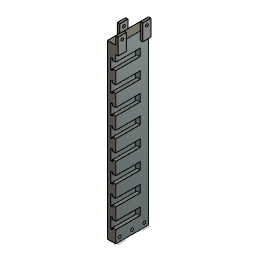
Stand v1 (Autodesk Fusion 360 design; units mm, degrees)
Autodesk Fusion 360 part; units mm, degrees
sketch "Sketch1" plane through (0, 0, 0) normal (0, 1, 0) x (1, 0, 0)
  line L0 (0, 0) -> (10, 0)
  line L1 (10, 0) -> (10, -40)
  line L2 (10, -40) -> (0, -40)
  line L3 (0, -40) -> (0, 0)
  dimension "d1" = 10
  dimension "d2" = 40
  constraint horizontal L0
  constraint vertical L1
  constraint horizontal L2
  constraint vertical L3
  constraint coincident L0.start L3.end
  measures "d1" distance of L1.end L2.end
  measures "d2" distance of L0.end L1.end
extrude "Extrude1" add sketch "Sketch1" along normal blind 210
sketch "Sketch2" plane through (0, 210, 0) normal (0, 1, 0) x (-1, 0, 0)
  line L0 (0, 40) -> (-10, 40)
  line L1 (-10, 40) -> (-10, 0)
  line L2 (-10, 0) -> (0, 0)
  line L3 (0, 0) -> (0, 40)
  line L4 (0, 15) -> (3, 15)
  line L5 (3, 15) -> (3, 25)
  line L6 (3, 25) -> (0, 25)
  line L7 (0, 25) -> (0, 15)
  line L8 (-10, 0) -> (-13, 0)
  line L9 (-13, 0) -> (-13, 10)
  line L10 (-13, 10) -> (-10, 10)
  line L11 (-10, 10) -> (-10, 0)
  line L12 (-10, 30) -> (-13, 30)
  line L13 (-13, 30) -> (-13, 40)
  line L14 (-13, 40) -> (-10, 40)
  line L15 (-10, 40) -> (-10, 30)
  dimension "d5" = 3
  dimension "d10" = 3
  dimension "d11" = 3
  constraint horizontal L4
  constraint vertical L5
  constraint horizontal L6
  constraint vertical L7
  constraint coincident L3 L4.start
  constraint horizontal L8
  constraint vertical L9
  constraint horizontal L10
  constraint vertical L11
  constraint coincident L1.end L2.start
  constraint horizontal L12
  constraint vertical L13
  constraint horizontal L14
  constraint vertical L15
  constraint coincident L1 L12.start
  measures "d5" distance of L5.end L6.end
  measures "d10" distance of L13.end L0.end
  measures "d11" distance of L1.end L8.end
extrude "Extrude2" add sketch "Sketch2" along normal blind 10 and the other way blind 10 contours L1 L12 L13 L14 L15 | L3 L4 L5 L6 L7 | L1 L8 L9 L10 L11
sketch "Sketch3" plane through (10, 0, 0) normal (1, 0, 0) x (0, 0, -1)
  line L0 (-10, 200) -> (-10, 210)
  line L1 (-10, 210) -> (-30, 210)
  line L2 (-30, 210) -> (-30, 200)
  line L3 (-30, 200) -> (-40, 200)
  line L4 (-40, 200) -> (-40, 0)
  line L5 (-40, 0) -> (0, 0)
  line L6 (0, 0) -> (0, 200)
  line L7 (0, 200) -> (-10, 200)
sketch "Sketch4" plane through (0, 0, 40) normal (0, 0, 1) x (1, 0, 0)
  line L0 (0, 0) -> (10, 0)
  line L1 (10, 0) -> (10, 200)
  line L2 (10, 200) -> (13, 200)
  line L3 (13, 200) -> (13, 220)
  line L4 (13, 220) -> (10, 220)
  line L5 (10, 220) -> (10, 210)
  line L6 (10, 210) -> (0, 210)
  line L7 (0, 210) -> (0, 0)
  line L8 (10, 15) -> (4, 15)
  line L9 (4, 15) -> (4, 20)
  line L10 (4, 20) -> (10, 20)
  line L11 (10, 20) -> (10, 15)
  line L12 (4, 20) -> (7, 20)
  line L13 (7, 20) -> (7, 22)
  line L14 (7, 22) -> (4, 22)
  line L15 (4, 22) -> (4, 20)
  line L16 (4, 22) -> (10, 22)
  line L17 (10, 22) -> (10, 24)
  line L18 (10, 24) -> (4, 24)
  line L19 (4, 24) -> (4, 22)
  line L20 (4, 44) -> (10, 44)
  line L21 (4, 46) -> (10, 46)
  line L22 (7, 44) -> (7, 46)
  line L23 (4, 46) -> (4, 44)
  line L24 (10, 48) -> (4, 48)
  line L25 (4, 39) -> (4, 44)
  line L26 (10, 39) -> (4, 39)
  line L27 (10, 44) -> (10, 39)
  line L28 (10, 46) -> (10, 48)
  line L29 (4, 48) -> (4, 46)
  line L30 (4, 68) -> (10, 68)
  line L31 (4, 70) -> (10, 70)
  line L32 (7, 68) -> (7, 70)
  line L33 (4, 70) -> (4, 68)
  line L34 (10, 72) -> (4, 72)
  line L35 (4, 63) -> (4, 68)
  line L36 (10, 63) -> (4, 63)
  line L37 (10, 68) -> (10, 63)
  line L38 (10, 70) -> (10, 72)
  line L39 (4, 72) -> (4, 70)
  line L40 (4, 92) -> (10, 92)
  line L41 (4, 94) -> (10, 94)
  line L42 (7, 92) -> (7, 94)
  line L43 (4, 94) -> (4, 92)
  line L44 (10, 96) -> (4, 96)
  line L45 (4, 87) -> (4, 92)
  line L46 (10, 87) -> (4, 87)
  line L47 (10, 92) -> (10, 87)
  line L48 (10, 94) -> (10, 96)
  line L49 (4, 96) -> (4, 94)
  line L50 (4, 116) -> (10, 116)
  line L51 (4, 118) -> (10, 118)
  line L52 (7, 116) -> (7, 118)
  line L53 (4, 118) -> (4, 116)
  line L54 (10, 120) -> (4, 120)
  line L55 (4, 111) -> (4, 116)
  line L56 (10, 111) -> (4, 111)
  line L57 (10, 116) -> (10, 111)
  line L58 (10, 118) -> (10, 120)
  line L59 (4, 120) -> (4, 118)
  line L60 (4, 140) -> (10, 140)
  line L61 (4, 142) -> (10, 142)
  line L62 (7, 140) -> (7, 142)
  line L63 (4, 142) -> (4, 140)
  line L64 (10, 144) -> (4, 144)
  line L65 (4, 135) -> (4, 140)
  line L66 (10, 135) -> (4, 135)
  line L67 (10, 140) -> (10, 135)
  line L68 (10, 142) -> (10, 144)
  line L69 (4, 144) -> (4, 142)
  line L70 (4, 164) -> (10, 164)
  line L71 (4, 166) -> (10, 166)
  line L72 (7, 164) -> (7, 166)
  line L73 (4, 166) -> (4, 164)
  line L74 (10, 168) -> (4, 168)
  line L75 (4, 159) -> (4, 164)
  line L76 (10, 159) -> (4, 159)
  line L77 (10, 164) -> (10, 159)
  line L78 (10, 166) -> (10, 168)
  line L79 (4, 168) -> (4, 166)
  line L80 (4, 188) -> (10, 188)
  line L81 (4, 190) -> (10, 190)
  line L82 (7, 188) -> (7, 190)
  line L83 (4, 190) -> (4, 188)
  line L84 (10, 192) -> (4, 192)
  line L85 (4, 183) -> (4, 188)
  line L86 (10, 183) -> (4, 183)
  line L87 (10, 188) -> (10, 183)
  line L88 (10, 190) -> (10, 192)
  line L89 (4, 192) -> (4, 190)
  dimension "d12" = 5
  dimension "d13" = 2
  dimension "d14" = 2
  dimension "d15" = 6
  dimension "d16" = 3
  dimension "d17" = 15
  dimension "d20" = 168
  dimension "d21" = 0
  constraint horizontal L8
  constraint vertical L9
  constraint horizontal L10
  constraint vertical L11
  constraint coincident L1 L8.start
  constraint horizontal L12
  constraint vertical L13
  constraint horizontal L14
  constraint vertical L15
  constraint horizontal L16
  constraint vertical L17
  constraint horizontal L18
  constraint vertical L19
  constraint coincident L1 L17.end
  measures "d12" distance of L8.end L9.end
  measures "d13" distance of L9.end L14.end
  measures "d14" distance of L14.end L18.end
  measures "d15" distance of L8.start L8.end
  measures "d16" distance of L13 L15
  measures "d17" distance of L0 L8
extrude "Extrude3" cut sketch "Sketch4" against normal blind 30 contours L1 L8 L9 L10 L11 L12 | L1 L10 L13 L16 | L1 L14 L16 L17 L18 L19 | L10 L12 L13 L14 L15 L16 | L1 L20 L25 L26 L27 | L1 L20 L21 L22 | L1 L81 L84 L88 L89 | L1 L21 L24 L28 L29 | L20 L21 L22 L23 | L1 L80 L81 L82 | L1 L80 L85 L86 L87 | L80 L81 L82 L83 | L1 L30 L35 L36 L37 | L1 L30 L31 L32 | L1 L71 L74 L78 L79 | L1 L31 L34 L38 L39 | L30 L31 L32 L33 | L1 L70 L71 L72 | L1 L70 L75 L76 L77 | L70 L71 L72 L73 | L1 L40 L45 L46 L47 | L1 L40 L41 L42 | L1 L61 L64 L68 L69 | L1 L41 L44 L48 L49 | L40 L41 L42 L43 | L1 L60 L61 L62 | L1 L60 L65 L66 L67 | L60 L61 L62 L63 | L1 L50 L55 L56 L57 | L1 L50 L51 L52 | L1 L51 L54 L58 L59 | L50 L51 L52 L53
sketch "Sketch6" plane through (0, 0, 40) normal (0, 0, 1) x (1, 0, 0)
  line L0 (4, 120) -> (10, 120)
  line L1 (10, 120) -> (10, 135)
  line L2 (10, 135) -> (4, 135)
  line L3 (4, 135) -> (4, 144)
  line L4 (4, 144) -> (10, 144)
  line L5 (10, 144) -> (10, 159)
  line L6 (10, 159) -> (4, 159)
  line L7 (4, 159) -> (4, 168)
  line L8 (4, 168) -> (10, 168)
  line L9 (10, 168) -> (10, 183)
  line L10 (10, 183) -> (4, 183)
  line L11 (4, 183) -> (4, 192)
  line L12 (4, 192) -> (10, 192)
  line L13 (10, 192) -> (10, 200)
  line L14 (10, 200) -> (13, 200)
  line L15 (13, 200) -> (13, 220)
  line L16 (13, 220) -> (10, 220)
  line L17 (10, 220) -> (10, 210)
  line L18 (10, 210) -> (0, 210)
  line L19 (0, 210) -> (0, 0)
  line L20 (0, 0) -> (10, 0)
  line L21 (10, 0) -> (10, 15)
  line L22 (10, 15) -> (4, 15)
  line L23 (4, 15) -> (4, 24)
  line L24 (4, 24) -> (10, 24)
  line L25 (10, 24) -> (10, 39)
  line L26 (10, 39) -> (4, 39)
  line L27 (4, 39) -> (4, 48)
  line L28 (4, 48) -> (10, 48)
  line L29 (10, 48) -> (10, 63)
  line L30 (10, 63) -> (4, 63)
  line L31 (4, 63) -> (4, 72)
  line L32 (4, 72) -> (10, 72)
  line L33 (10, 72) -> (10, 87)
  line L34 (10, 87) -> (4, 87)
  line L35 (4, 87) -> (4, 96)
  line L36 (4, 96) -> (10, 96)
  line L37 (10, 96) -> (10, 111)
  line L38 (10, 111) -> (4, 111)
  line L39 (4, 111) -> (4, 120)
  line L40 (4, 192) -> (6, 192)
  line L41 (6, 192) -> (6, 194)
  line L42 (6, 194) -> (4, 194)
  line L43 (4, 194) -> (4, 192)
  line L44 (4, 183) -> (6, 183)
  line L45 (6, 183) -> (6, 181)
  line L46 (6, 181) -> (4, 181)
  line L47 (4, 181) -> (4, 183)
  line L48 (6, 157) -> (4, 157)
  line L49 (6, 159) -> (6, 157)
  line L50 (4, 159) -> (6, 159)
  line L51 (4, 157) -> (4, 159)
  line L52 (4, 168) -> (6, 168)
  line L53 (6, 168) -> (6, 170)
  line L54 (6, 170) -> (4, 170)
  line L55 (4, 170) -> (4, 168)
  line L56 (6, 133) -> (4, 133)
  line L57 (6, 135) -> (6, 133)
  line L58 (4, 135) -> (6, 135)
  line L59 (4, 133) -> (4, 135)
  line L60 (4, 144) -> (6, 144)
  line L61 (6, 144) -> (6, 146)
  line L62 (6, 146) -> (4, 146)
  line L63 (4, 146) -> (4, 144)
  line L64 (6, 109) -> (4, 109)
  line L65 (6, 111) -> (6, 109)
  line L66 (4, 111) -> (6, 111)
  line L67 (4, 109) -> (4, 111)
  line L68 (4, 120) -> (6, 120)
  line L69 (6, 120) -> (6, 122)
  line L70 (6, 122) -> (4, 122)
  line L71 (4, 122) -> (4, 120)
  line L72 (6, 85) -> (4, 85)
  line L73 (6, 87) -> (6, 85)
  line L74 (4, 87) -> (6, 87)
  line L75 (4, 85) -> (4, 87)
  line L76 (4, 96) -> (6, 96)
  line L77 (6, 96) -> (6, 98)
  line L78 (6, 98) -> (4, 98)
  line L79 (4, 98) -> (4, 96)
  line L80 (6, 61) -> (4, 61)
  line L81 (6, 63) -> (6, 61)
  line L82 (4, 63) -> (6, 63)
  line L83 (4, 61) -> (4, 63)
  line L84 (4, 72) -> (6, 72)
  line L85 (6, 72) -> (6, 74)
  line L86 (6, 74) -> (4, 74)
  line L87 (4, 74) -> (4, 72)
  line L88 (6, 37) -> (4, 37)
  line L89 (6, 39) -> (6, 37)
  line L90 (4, 39) -> (6, 39)
  line L91 (4, 37) -> (4, 39)
  line L92 (4, 48) -> (6, 48)
  line L93 (6, 48) -> (6, 50)
  line L94 (6, 50) -> (4, 50)
  line L95 (4, 50) -> (4, 48)
  line L96 (6, 13) -> (4, 13)
  line L97 (6, 15) -> (6, 13)
  line L98 (4, 15) -> (6, 15)
  line L99 (4, 13) -> (4, 15)
  line L100 (4, 24) -> (6, 24)
  line L101 (6, 24) -> (6, 26)
  line L102 (6, 26) -> (4, 26)
  line L103 (4, 26) -> (4, 24)
  dimension "d31" = 2
  dimension "d32" = 2
  dimension "d33" = 2
  dimension "d34" = 2
  dimension "d37" = -168
  dimension "d38" = 0
  constraint horizontal L40
  constraint vertical L41
  constraint horizontal L42
  constraint vertical L43
  constraint coincident L11.end L12.start
  constraint horizontal L44
  constraint vertical L45
  constraint horizontal L46
  constraint vertical L47
  constraint coincident L10.end L11.start
  measures "d31" distance of L45.end L46.end
  measures "d32" distance of L44.end L45.end
  measures "d33" distance of L11.end L42.end
  measures "d34" distance of L41.end L42.end
extrude "Extrude5" cut sketch "Sketch6" against normal blind 30 contours L0 L68 L69 L70 L71 | L38 L64 L65 L66 L67 | L2 L56 L57 L58 L59 | L36 L76 L77 L78 L79 | L4 L60 L61 L62 L63 | L34 L72 L73 L74 L75 | L6 L48 L49 L50 L51 | L32 L84 L85 L86 L87 | L8 L52 L53 L54 L55 | L30 L80 L81 L82 L83 | L10 L44 L45 L46 L47 | L28 L92 L93 L94 L95 | L12 L40 L41 L42 L43 | L26 L88 L89 L90 L91 | L24 L100 L101 L102 L103 | L22 L96 L97 L98 L99
sketch "Sketch7" plane through (13, 0, 0) normal (1, 0, 0) x (0, 0, -1)
  line L0 (-30, 200) -> (-30, 220)
  line L1 (-30, 220) -> (-40, 220)
  line L2 (-40, 220) -> (-40, 200)
  line L3 (-40, 200) -> (-30, 200)
  circle A0 centre (-35, 215) radius 1.7
  circle A1 centre (-5, 215) radius 1.7
  circle A2 centre (-20, 215) radius 1.7
  line L4 (-35, 220) -> (-35, 200) construction
  line L5 (-5, 220) -> (-5, 200) construction
  line L6 (-20, 220) -> (-20, 210) construction
  line L7 (-25, 220) -> (-15, 220)
  line L8 (-10, 220) -> (0, 220)
  dimension "d41" = 3.4
  dimension "d42" = 3.4
  dimension "d43" = 3.4
  dimension "d44" = 5
  dimension "d45" = 5
  dimension "d46" = 5
  constraint midpoint L1 L4.start
  constraint midpoint L3 L4.end
  constraint perpendicular L3 L5
  constraint vertical L6
  constraint coincident A0.centre L4
  constraint coincident A2.centre L6
  constraint coincident A1.centre L5
  measures "d41" diameter of A0
  measures "d42" diameter of A1
  measures "d43" diameter of A2
  measures "d44" distance of A2.centre L7
  measures "d45" distance of A1.centre L8
  measures "d46" distance of L1 A0.centre
extrude "Extrude6" cut sketch "Sketch7" against normal blind 40 contours A0 | A1 | A2
sketch "Sketch8" plane through (10, 0, 0) normal (1, 0, 0) x (0, 0, -1)
  circle A0 centre (-35, 5) radius 1.7
  circle A1 centre (-20, 5) radius 1.7
  circle A2 centre (-5, 5) radius 1.7
  line L0 (-40, 0) -> (0, 0)
  line L1 (-40, 200) -> (-40, 0)
  line L2 (0, 0) -> (0, 200)
  dimension "d49" = 3.4
  dimension "d50" = 3.4
  dimension "d51" = 3.4
  dimension "d52" = 5
  dimension "d53" = 5
  dimension "d54" = 5
  dimension "d55" = 5
  dimension "d56" = 5
  dimension "d57" = 20
  measures "d49" diameter of A0
  measures "d50" diameter of A1
  measures "d51" diameter of A2
  measures "d52" distance of A0.centre L0
  measures "d53" distance of A1.centre L0
  measures "d54" distance of A2.centre L0
  measures "d55" distance of A0.centre L1
  measures "d56" distance of A2.centre L2
  measures "d57" distance of A1.centre L2
extrude "Extrude7" cut sketch "Sketch8" against normal blind 37
